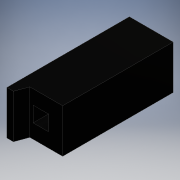
# Autodesk Inventor part: body
Saved by Autodesk Inventor 2016 (Build 200138000, 138)
## iProperties
Created: 2016-08-01
Part Number: body
Material: Generic
Document SubType Name: Modeling
Designer: Jonathan
Density: 1 g/cm^3
Appearance: Smooth - Black
Author: Jonathan
Autodesk Inventor part; units mm, degrees
ref_plane "YZ Plane" through (0, 0, 0) normal (1, 0, 0) x (0, 1, 0)
ref_plane "XZ Plane" through (0, 0, 0) normal (0, 1, 0) x (-1, 0, 0)
ref_plane "XY Plane" through (0, 0, 0) normal (0, 0, 1) x (1, 0, 0)
sketch "Sketch6" plane through (0, 0, 0) normal (0, 0, 1) x (1, 0, 0)
  line L0 (-2.54, 6.4141) -> (0, 6.4141)
  line L1 (0, 6.4141) -> (0, 0)
  line L2 (0, 0) -> (-1.905, 0)
  line L3 (-1.905, 0) -> (-2.159, -0.6979)
  line L4 (-2.159, -0.6979) -> (-2.54, -0.6979)
  line L5 (-2.54, -0.6979) -> (-2.54, 6.4141)
  dimension "d25" = 2.54
  dimension "d26" = 7.112
  dimension "d27" = 110
  dimension "d28" = 1.905
  dimension "d29" = 0.381
  constraints: 12 end point, 2 perpendicular, 1 coincident, 1 horizontal, 1 parallel, 1 vertical
  measures "d25" distance of L0.start L0.end
  measures "d26" distance of L4.end L0.start
  measures "d27" angle of L4 L3
  measures "d28" distance of L1.end L2.end
  measures "d29" distance of L3.end L4.end
extrude "Extrusion3" add sketch "Sketch6" along normal mid plane 2.54
sketch "Sketch7" plane through (-2.54, 6.4141, -1.27) normal (0, 1, 0) x (1, 0, 0)
  line L0 (0.8255, -0.8255) -> (1.7145, -0.8255)
  line L1 (1.7145, -0.8255) -> (1.7145, -1.7145)
  line L2 (1.7145, -1.7145) -> (0.8255, -1.7145)
  line L3 (0.8255, -1.7145) -> (0.8255, -0.8255)
  line L4 (0.8255, -0.8255) -> (1.7145, -1.7145) construction
  line L5 (1.7145, -0.8255) -> (0.8255, -1.7145) construction
  line L6 (2.54, -2.54) -> (2.54, 0) projected
  line L7 (0, 0) -> (2.54, 0) projected
  point P0 (1.27, -1.27)
  point P1 (1.27, -1.27)
  point P2 (1.27, -1.27)
  point P3 (2.54, -1.27)
  point P4 (1.27, 0)
  dimension "d32" = 0.889
  constraints: 12 end point, 6 midpoint, 2 parallel, 2 perpendicular, 1 horizontal, 1 horizontal alignment, 1 vertical alignment
  measures "d32" distance of L0.start L0.end
extrude "Extrusion4" cut sketch "Sketch7" against normal through all
chamfer "Chamfer2" distance 0.381 angle 45 4 edges at (-1.27, 6.4141, -0.4445) (-1.7145, 6.4141, 0) (-1.27, 6.4141, 0.4445) (-0.8255, 6.4141, 0)
body "Solid2"
